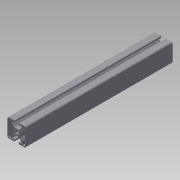
# Autodesk Inventor part: 1504-LS
Saved by Autodesk Inventor 2013 (Build 170138000, 138)
## iProperties
Created: 2014-04-23
Part Number: 1504-LS
Material: Generic
Document SubType Name: Modeling
Density: 1 g/cm^3
Vendor: 80/20 Inc.
Engineer: Ross Bowman
Designer: Ross Bowman
Catalog Web Link: 8020.net
Company: 80/20 Inc.
Author: Ross Bowman
Keywords: 80/20 , 8020 , T-Slot , Extrusion
Material: 6105-T5 Aluminum
Autodesk Inventor part; units mm, degrees
ref_plane "YZ Plane" through (0, 0, 0) normal (1, 0, 0) x (0, 1, 0)
ref_plane "XZ Plane" through (0, 0, 0) normal (0, 1, 0) x (-1, 0, 0)
ref_plane "XY Plane" through (0, 0, 0) normal (0, 0, 1) x (1, 0, 0)
sketch "Sketch1" plane through (0, 0, 0) normal (0, 0, 1) x (1, 0, 0)
  arc A0 (17.2478, 14.452) -> (14.4539, 17.2462) centre (14.4538, 14.4522) ccw
  line L0 (17.2463, -14.4523) -> (17.2478, 14.452)
  arc A1 (14.4525, -17.2462) -> (17.2463, -14.4523) centre (14.4523, -14.4522) ccw
  line L1 (12.5802, -17.2463) -> (14.4525, -17.2462)
  arc A2 (12.1992, -16.8653) -> (12.5802, -17.2463) centre (12.5802, -16.8653) ccw
  line L2 (12.1994, -11.3582) -> (12.1992, -16.8653)
  arc A3 (12.1994, -11.3582) -> (11.2694, -9.1129) centre (9.0244, -11.3581) ccw
  line L3 (8.2571, -6.1009) -> (11.2694, -9.1129)
  arc A4 (6.8657, -2.742) -> (8.2571, -6.1009) centre (11.6155, -2.7421) ccw
  line L4 (6.8657, 2.742) -> (6.8657, -2.742)
  arc A5 (8.2571, 6.1009) -> (6.8657, 2.742) centre (11.6155, 2.7421) ccw
  line L5 (11.2694, 9.1129) -> (8.2571, 6.1009)
  arc A6 (11.2694, 9.1129) -> (12.1994, 11.3582) centre (9.0244, 11.3581) ccw
  line L6 (12.1992, 16.8653) -> (12.1994, 11.3582)
  arc A7 (12.5802, 17.2463) -> (12.1992, 16.8653) centre (12.5802, 16.8653) ccw
  line L7 (14.4539, 17.2462) -> (12.5802, 17.2463)
  arc A8 (-17.2463, -14.4523) -> (-14.4525, -17.2462) centre (-14.4523, -14.4522) ccw
  line L8 (-17.2478, 14.452) -> (-17.2463, -14.4523)
  arc A9 (-14.4539, 17.2462) -> (-17.2478, 14.452) centre (-14.4538, 14.4522) ccw
  line L9 (-12.5802, 17.2463) -> (-14.4539, 17.2462)
  arc A10 (-12.1992, 16.8653) -> (-12.5802, 17.2463) centre (-12.5802, 16.8653) ccw
  line L10 (-12.1994, 11.3582) -> (-12.1992, 16.8653)
  arc A11 (-12.1994, 11.3582) -> (-11.2694, 9.1129) centre (-9.0244, 11.3581) ccw
  line L11 (-8.2571, 6.1009) -> (-11.2694, 9.1129)
  arc A12 (-6.8657, 2.742) -> (-8.2571, 6.1009) centre (-11.6155, 2.7421) ccw
  line L12 (-6.8657, -2.742) -> (-6.8657, 2.742)
  arc A13 (-8.2571, -6.1009) -> (-6.8657, -2.742) centre (-11.6155, -2.7421) ccw
  line L13 (-11.2694, -9.1129) -> (-8.2571, -6.1009)
  arc A14 (-11.2694, -9.1129) -> (-12.1994, -11.3582) centre (-9.0244, -11.3581) ccw
  line L14 (-12.1992, -16.8653) -> (-12.1994, -11.3582)
  arc A15 (-12.5802, -17.2463) -> (-12.1992, -16.8653) centre (-12.5802, -16.8653) ccw
  line L15 (-14.4525, -17.2462) -> (-12.5802, -17.2463)
  arc A16 (2.7269, -4.3433) -> (4.3433, -2.7269) centre (3.5351, -3.5351) ccw
  line L16 (1.3564, -2.9729) -> (2.7269, -4.3433)
  arc A17 (-1.3564, -2.9729) -> (1.3564, -2.9729) centre (0, 0) ccw
  line L17 (-2.7269, -4.3433) -> (-1.3564, -2.9729)
  arc A18 (-4.3433, -2.7269) -> (-2.7269, -4.3433) centre (-3.5351, -3.5351) ccw
  line L18 (-2.9729, -1.3564) -> (-4.3433, -2.7269)
  arc A19 (-2.9729, 1.3564) -> (-2.9729, -1.3564) centre (0, 0) ccw
  line L19 (-4.3433, 2.7269) -> (-2.9729, 1.3564)
  arc A20 (-2.7269, 4.3433) -> (-4.3433, 2.7269) centre (-3.5351, 3.5351) ccw
  line L20 (-1.3564, 2.9729) -> (-2.7269, 4.3433)
  arc A21 (1.3564, 2.9729) -> (-1.3564, 2.9729) centre (0, 0) ccw
  line L21 (2.7269, 4.3433) -> (1.3564, 2.9729)
  arc A22 (4.3433, 2.7269) -> (2.7269, 4.3433) centre (3.5351, 3.5351) ccw
  line L22 (2.9729, 1.3564) -> (4.3433, 2.7269)
  arc A23 (2.9729, -1.3564) -> (2.9729, 1.3564) centre (0, 0) ccw
  line L23 (4.3433, -2.7269) -> (2.9729, -1.3564)
  arc A24 (19.05, 15.875) -> (15.875, 19.05) centre (15.875, 15.875) ccw
  line L24 (15.875, 19.05) -> (5.6388, 19.05)
  arc A25 (5.6388, 19.05) -> (4.064, 17.4752) centre (5.6388, 17.4752) ccw
  line L25 (4.064, 17.4752) -> (4.064, 16.5608)
  arc A26 (4.064, 16.5608) -> (5.6388, 14.986) centre (5.6388, 16.5608) ccw
  line L26 (5.6388, 14.986) -> (6.477, 14.986)
  arc A27 (6.477, 14.986) -> (6.858, 15.367) centre (6.477, 15.367) ccw
  line L27 (6.858, 15.367) -> (6.858, 15.4432)
  arc A28 (7.239, 15.8242) -> (6.858, 15.4432) centre (7.239, 15.4432) ccw
  line L28 (7.239, 15.8242) -> (9.017, 15.8242)
  arc A29 (10.287, 14.5542) -> (9.017, 15.8242) centre (9.017, 14.5542) ccw
  line L29 (10.287, 14.5542) -> (10.287, 12.9683)
  arc A30 (9.915, 12.0703) -> (10.287, 12.9683) centre (9.017, 12.9683) ccw
  line L30 (9.915, 12.0703) -> (5.9669, 8.1222)
  arc A31 (2.6083, 6.731) -> (5.9669, 8.1222) centre (2.6083, 11.4808) ccw
  line L31 (2.6083, 6.731) -> (-2.6083, 6.731)
  arc A32 (-5.9669, 8.1222) -> (-2.6083, 6.731) centre (-2.6083, 11.4808) ccw
  line L32 (-5.9669, 8.1222) -> (-9.915, 12.0703)
  arc A33 (-10.287, 12.9683) -> (-9.915, 12.0703) centre (-9.017, 12.9683) ccw
  line L33 (-10.287, 12.9683) -> (-10.287, 14.5542)
  arc A34 (-9.017, 15.8242) -> (-10.287, 14.5542) centre (-9.017, 14.5542) ccw
  line L34 (-9.017, 15.8242) -> (-7.239, 15.8242)
  arc A35 (-6.858, 15.4432) -> (-7.239, 15.8242) centre (-7.239, 15.4432) ccw
  line L35 (-6.858, 15.4432) -> (-6.858, 15.367)
  arc A36 (-6.858, 15.367) -> (-6.477, 14.986) centre (-6.477, 15.367) ccw
  line L36 (-6.477, 14.986) -> (-5.6388, 14.986)
  arc A37 (-5.6388, 14.986) -> (-4.064, 16.5608) centre (-5.6388, 16.5608) ccw
  line L37 (-4.064, 16.5608) -> (-4.064, 17.4752)
  arc A38 (-4.064, 17.4752) -> (-5.6388, 19.05) centre (-5.6388, 17.4752) ccw
  line L38 (-5.6388, 19.05) -> (-15.875, 19.05)
  arc A39 (-15.875, 19.05) -> (-19.05, 15.875) centre (-15.875, 15.875) ccw
  line L39 (-19.05, 15.875) -> (-19.05, -15.875)
  arc A40 (-19.05, -15.875) -> (-15.875, -19.05) centre (-15.875, -15.875) ccw
  line L40 (-15.875, -19.05) -> (-5.6388, -19.05)
  arc A41 (-5.6388, -19.05) -> (-4.064, -17.4752) centre (-5.6388, -17.4752) ccw
  line L41 (-4.064, -17.4752) -> (-4.064, -16.5608)
  arc A42 (-4.064, -16.5608) -> (-5.6388, -14.986) centre (-5.6388, -16.5608) ccw
  line L42 (-5.6388, -14.986) -> (-6.477, -14.986)
  arc A43 (-6.477, -14.986) -> (-6.858, -15.367) centre (-6.477, -15.367) ccw
  line L43 (-6.858, -15.367) -> (-6.858, -15.4432)
  arc A44 (-7.239, -15.8242) -> (-6.858, -15.4432) centre (-7.239, -15.4432) ccw
  line L44 (-7.239, -15.8242) -> (-9.017, -15.8242)
  arc A45 (-10.287, -14.5542) -> (-9.017, -15.8242) centre (-9.017, -14.5542) ccw
  line L45 (-10.287, -14.5542) -> (-10.287, -12.9683)
  arc A46 (-9.915, -12.0703) -> (-10.287, -12.9683) centre (-9.017, -12.9683) ccw
  line L46 (-9.915, -12.0703) -> (-5.9669, -8.1222)
  arc A47 (-2.6083, -6.731) -> (-5.9669, -8.1222) centre (-2.6083, -11.4808) ccw
  line L47 (-2.6083, -6.731) -> (2.6083, -6.731)
  arc A48 (5.9669, -8.1222) -> (2.6083, -6.731) centre (2.6083, -11.4808) ccw
  line L48 (5.9669, -8.1222) -> (9.915, -12.0703)
  arc A49 (10.287, -12.9683) -> (9.915, -12.0703) centre (9.017, -12.9683) ccw
  line L49 (10.287, -12.9683) -> (10.287, -14.5542)
  arc A50 (9.017, -15.8242) -> (10.287, -14.5542) centre (9.017, -14.5542) ccw
  line L50 (9.017, -15.8242) -> (7.239, -15.8242)
  arc A51 (6.858, -15.4432) -> (7.239, -15.8242) centre (7.239, -15.4432) ccw
  line L51 (6.858, -15.4432) -> (6.858, -15.367)
  arc A52 (6.858, -15.367) -> (6.477, -14.986) centre (6.477, -15.367) ccw
  line L52 (6.477, -14.986) -> (5.6388, -14.986)
  arc A53 (5.6388, -14.986) -> (4.064, -16.5608) centre (5.6388, -16.5608) ccw
  line L53 (4.064, -16.5608) -> (4.064, -17.4752)
  arc A54 (4.064, -17.4752) -> (5.6388, -19.05) centre (5.6388, -17.4752) ccw
  line L54 (5.6388, -19.05) -> (15.875, -19.05)
  arc A55 (15.875, -19.05) -> (19.05, -15.875) centre (15.875, -15.875) ccw
  line L55 (19.05, -15.875) -> (19.05, 15.875)
  constraints: 112 end point, 112 point on circle, 56 centre point
extrude "Extrusion1" add sketch "Sketch1" against normal blind 304.8
body "Solid1"
